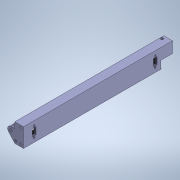
# Autodesk Inventor part: slide rail
Saved by Autodesk Inventor 2020 (Build 240168000, 168)
## iProperties
Created: 2026-07-07
Part Number: slide rail
Material: Steel
Document SubType Name: Modeling
Designer: drago
Density: 7.85 g/cm^3
Appearance: Slate Blue
Author: drago
Autodesk Inventor part; units mm, degrees
ref_plane "YZ Plane" through (0, 0, 0) normal (1, 0, 0) x (0, 1, 0)
ref_plane "XZ Plane" through (0, 0, 0) normal (0, 1, 0) x (-1, 0, 0)
ref_plane "XY Plane" through (0, 0, 0) normal (0, 0, 1) x (1, 0, 0)
sketch "Sketch1" plane through (0, 0, 0) normal (0, 0, 1) x (1, 0, 0)
  line L0 (-0.5, -2.9) -> (6.5, -2.9)
  line L1 (6.5, -2.9) -> (6.5, 12.9)
  line L2 (6.5, 12.9) -> (-0.5, 12.9)
  line L3 (-0.5, 14.9) -> (8.5, 14.9)
  line L4 (8.5, 14.9) -> (8.5, -4.9)
  line L5 (8.5, -4.9) -> (-0.5, -4.9)
  line L6 (-0.5, 12.9) -> (-0.5, 14.9)
  line L7 (-0.5, -4.9) -> (-0.5, -2.9)
  circle A0 centre (-5, 5) radius 1.45
  circle A1 centre (-5, 5) radius 1.45
  circle A2 centre (-5, 5) radius 4
  point P0 (0, 0)
  constraints: 16 end point, 3 centre point, 3 perpendicular, 2 coincident, 2 parallel, 1 horizontal, 2 other
extrude "Extrusion1" add sketch "Sketch1" along normal blind 180
extrude "Extrusion2" cut sketch "Sketch1" along normal blind 160 contours A2
extrude "Extrusion3" add sketch "Sketch1" along normal blind 20 contours A2
sketch "Sketch2" plane through (-0.5, 14.9, 0) normal (0, 1, 0) x (1, 0, 0)
  line L0 (9, 0) -> (0, 0) projected
  line L1 (0, 0) -> (0, -180) projected
  line L2 (9, -180) -> (0, -180) projected
  line L3 (9, 0) -> (9, -180) projected
  point P0 (0.5, 0)
extrude "Extrusion4" add sketch "Sketch2" along normal blind 1
sketch "Sketch3" plane through (-0.5, -4.9, 0) normal (0, -1, 0) x (1, 0, 0)
  line L0 (0, 0) -> (9, 0) projected
  line L1 (9, 0) -> (9, 180) projected
  line L2 (0, 180) -> (9, 180) projected
  line L3 (0, 0) -> (0, 180) projected
  point P0 (0.5, 0)
extrude "Extrusion5" add sketch "Sketch3" along normal blind 1
sketch "Sketch4" plane through (8.5, 15.9, 180) normal (1, 0, 0) x (0, 0, -1)
  line L0 (180, 0) -> (180, -21.8) projected
  line L1 (0, 0) -> (180, 0) projected
  line L2 (0, 0) -> (0, -21.8) projected
  line L3 (180, -21.8) -> (0, -21.8) projected
  point P0 (180, -15.9)
extrude "Extrusion6" add sketch "Sketch4" along normal blind 1
sketch "Sketch5" plane through (-5, 5, 0) normal (0, 0, -1) x (-1, 0, 0)
  circle A0 centre (0, 0) radius 1.45 projected
  point P0 (-5, -5)
extrude "Extrusion7" add sketch "Sketch5" against normal blind 14
sketch "Sketch6" plane through (-5, 5, 180) normal (0, 0, 1) x (1, 0, 0)
  circle A0 centre (0, 0) radius 1.45 projected
  point P0 (5, -5)
extrude "Extrusion8" add sketch "Sketch6" against normal blind 14
sketch "Sketch7" plane through (-5, 5, 0) normal (0, 0, -1) x (-1, 0, 0)
  line L0 (-4.5, 7.9) -> (-4.5, 10.9) projected
  line L1 (-4.5, 10.9) -> (2.9603, 2.69)
  circle A0 centre (0, 0) radius 4 projected
  line L2 (-4.5, -7.9) -> (-4.5, -10.9) projected
  line L3 (-4.5, -10.9) -> (2.9603, -2.69)
  line L4 (-4.5, 7.9) -> (-11.5, 7.9) projected
  line L5 (-4.5, -7.9) -> (-4.5, -10.9) projected
  line L6 (-11.5, -7.9) -> (-4.5, -7.9) projected
  line L7 (-11.5, 7.9) -> (-11.5, -7.9) projected
  line L8 (-4.5, 7.9) -> (-11.5, 7.9) projected
  line L9 (-4.5, 7.9) -> (-4.5, 10.9) projected
  line L10 (-4.5, 10.9) -> (-14.5, 10.9) projected
  line L11 (-14.5, -10.9) -> (-14.5, 10.9) projected
  line L12 (-4.5, -10.9) -> (-14.5, -10.9) projected
  point P0 (-5, -5)
  point P1 (2.9603, -2.69)
  constraints: 4 end point, 4 other
extrude "Extrusion9" add sketch "Sketch7" against normal blind 18 contours L0 L1 A0 L3 L2 L6 L7 L4
sketch "Sketch8" plane through (-0.5, 12.9, 18) normal (-1, 0, 0) x (0, 0, 1)
  line L0 (0, 3) -> (0, 0) projected
  line L1 (0, 3) -> (-5, 3)
  line L2 (-5, 3) -> (-5, -3.9)
  line L3 (-5, -3.9) -> (0, -3.9)
  line L4 (0, -3.9) -> (0, 3)
  point P0 (-18, -12.9)
  dimension "d19" = 5
  constraints: 8 end point, 2 parallel, 1 horizontal, 1 perpendicular
  measures "d19" distance of L3.end L2.end
extrude "Extrusion10" cut sketch "Sketch8" along normal blind 18
sketch "Sketch9" plane through (-5, 5, 180) normal (0, 0, 1) x (1, 0, 0)
  line L0 (4.5, -7.9) -> (4.5, -10.9) projected
  line L1 (4.5, -10.9) -> (-2.9603, -2.69)
  arc A0 (0, 4) -> (-2.9603, 2.69) centre (0, 0) ccw projected
  line L2 (4.5, 10.9) -> (-2.9603, 2.69)
  line L3 (4.5, 7.9) -> (4.5, 4) projected
  line L4 (4.5, 4) -> (0, 4) projected
  arc A1 (-2.9603, -2.69) -> (0, 4) centre (0, 0) ccw projected
  line L5 (-2.9603, -2.69) -> (4.5, -10.9) projected
  line L6 (4.5, -7.9) -> (4.5, -10.9) projected
  line L7 (11.5, -7.9) -> (4.5, -7.9) projected
  line L8 (11.5, 7.9) -> (11.5, -7.9) projected
  line L9 (4.5, 7.9) -> (11.5, 7.9) projected
  line L10 (-1.77, 4) -> (4.5, 10.9) projected
  line L11 (4.5, 7.9) -> (4.5, 10.9) projected
  point P0 (5, -5)
  constraints: 4 end point, 1 tangent
extrude "Extrusion11" add sketch "Sketch9" against normal blind 18
sketch "Sketch10" plane through (-0.5, 9, 13) normal (-1, 0, 0) x (0, 0, 1)
  line L0 (149, 3.9) -> (149, 6.9) projected
  line L1 (149, 6.9) -> (154, 6.9)
  line L2 (154, 6.9) -> (154, 0)
  line L3 (154, 0) -> (149, 0)
  line L4 (149, 0) -> (149, 6.9)
  point P0 (-13, -9)
  dimension "d24" = 5
  constraints: 8 end point, 2 parallel, 1 horizontal, 1 perpendicular
  measures "d24" distance of L2.end L3.end
extrude "Extrusion12" cut sketch "Sketch10" along normal blind 18
sketch "Sketch12" plane through (-0.5, -5.9, 0) normal (0, -1, 0) x (1, 0, 0)
  line L0 (-5.95, 20) -> (-3.05, 20) projected
  circle A0 centre (2, 4) radius 1.4
  circle A1 centre (2, 4) radius 9.5
  point P0 (0.5, 0)
  dimension "d42" = 19
  constraints: 2 centre point, 1 coincident
  measures "d42" diameter of A1
extrude "Extrusion13" cut sketch "Sketch12" against normal blind 9
extrude "Extrusion14" cut sketch "Sketch12" against normal blind 23 contours A0
sketch "Sketch13" plane through (-0.5, 9, 13) normal (-1, 0, 0) x (0, 0, 1)
  line L0 (149, 0) -> (149, 3.9) projected
  line L1 (149, 0) -> (153.7, 0)
  line L2 (149, 3.2) -> (149, 0)
  line L3 (-13, 6.9) -> (167, 6.9) projected
  line L4 (149, 0) -> (159, 0)
  line L5 (159, 0) -> (159, 6.9)
  line L6 (159, 6.9) -> (149, 6.9)
  line L7 (149, 6.9) -> (149, 0)
  line L8 (5, 3.9) -> (5, 0) projected
  line L9 (5, 0) -> (-5, 0)
  line L10 (-5, 0) -> (-5, 6.9)
  line L11 (-5, 6.9) -> (5, 6.9)
  line L12 (5, 6.9) -> (5, 0)
  line L13 (5, 0) -> (0.3, 0)
  line L14 (5, 3.2) -> (5, 0)
  circle A0 centre (2.3, 3.2) radius 0.9
  circle A1 centre (151.7, 3.2) radius 0.9
  point P0 (-13, -9)
  point P1 (153.7, 0)
  dimension "d49" = 10
  dimension "d50" = 10
  constraints: 24 end point, 4 horizontal, 4 parallel, 2 centre point, 2 perpendicular, 2 point on line
  measures "d49" distance of L6.end L5.end
  measures "d50" distance of L10.end L11.end
extrude "Extrusion15" cut sketch "Sketch13" along normal blind 10 contours L0 L7 L3 L5 L4 L1 | L3 L12 L8 L9 L10 | A0 | A1
sketch "Sketch14" plane through (9.5, 15.9, 180) normal (1, 0, 0) x (0, 0, -1)
  line L0 (0, -21.8) -> (170.8765, -21.8) projected
  line L1 (0, 0) -> (8, 0)
  line L2 (8, 0) -> (8, -21.8)
  line L3 (8, -21.8) -> (0, -21.8)
  line L4 (0, -21.8) -> (0, 0)
  point P0 (180, -15.9)
  dimension "d60" = 8
  constraints: 8 end point, 2 parallel, 1 horizontal, 1 perpendicular, 1 point on line
  measures "d60" distance of L2.end L3.end
extrude "Extrusion17" cut sketch "Sketch14" against normal blind 20
sketch "Sketch15" plane through (9.5, -5.9, 172) normal (0, 0, 1) x (1, 0, 0)
  circle A0 centre (-14.5, 10.9) radius 1.45 projected
  circle A1 centre (-14.5, 10.9) radius 1.45
  point P0 (-9.5, 5.9)
  constraints: 1 centre point, 1 coincident
extrude "Extrusion18" cut sketch "Sketch15" against normal blind 20
sketch "Sketch16" plane through (-0.5, 3.1, 0) normal (0, -1, 0) x (1, 0, 0)
  line L0 (-8.5, 0) -> (-8.5, 20) projected
  line L1 (-8.5, 0) -> (-1.5, 0)
  line L2 (-1.5, 0) -> (-1.5, 10)
  line L3 (-1.5, 10) -> (-8.5, 10)
  line L4 (-8.5, 10) -> (-8.5, 0)
  point P0 (0.5, 0)
  dimension "d65" = 7
  dimension "d66" = 10
  constraints: 8 end point, 2 parallel, 1 horizontal, 1 perpendicular, 1 point on line
  measures "d65" distance of L3.end L2.end
  measures "d66" distance of L2.end L1.end
extrude "Extrusion19" cut sketch "Sketch16" along normal mid plane 30
sketch "Sketch17" plane through (-2, 3.1, 10) normal (0, 0, -1) x (-1, 0, 0)
  circle A0 centre (3, 1.9) radius 1.45 projected
  circle A1 centre (3, 1.9) radius 1.45
  point P0 (-2, -3.1)
  constraints: 1 centre point, 1 coincident
extrude "Extrusion20" cut sketch "Sketch17" against normal blind 30
sketch "Sketch18" plane through (-2, 3.1, 10) normal (0, 0, -1) x (-1, 0, 0)
  line L0 (0, 5.9) -> (0, 0) projected
  line L1 (0, 5.9) -> (8.7441, 5.9)
  line L2 (8.7441, 5.9) -> (8.7441, -5.7339)
  line L3 (8.7441, -5.7339) -> (0, -5.7339)
  line L4 (0, -5.7339) -> (0, 5.9)
  point P0 (-2, -3.1)
  constraints: 8 end point, 2 parallel, 1 horizontal, 1 perpendicular
extrude "Extrusion21" cut sketch "Sketch18" against normal blind 2
fillet "Fillet1" radius 2 1 edges at (9.5, -1.4, 9.1235)
sketch "Sketch19" plane through (9.5, -5.9, 172) normal (0, 0, 1) x (1, 0, 0)
  circle A0 centre (-14.5, 10.9) radius 1.45 projected
  circle A1 centre (-14.5, 10.9) radius 4
  line L0 (-10, 14.9) -> (-16.27, 14.9) projected
  line L1 (-16.27, 14.9) -> (-17.4603, 13.59)
  line L2 (-17.4603, 13.59) -> (-16.27, 14.9) projected
  point P0 (-9.5, 5.9)
  point P1 (-14.5, 14.9)
  constraints: 2 end point, 1 coincident, 1 collinear, 1 horizontal, 1 point on line, 3 other
extrude "Extrusion22" cut sketch "Sketch19" against normal blind 300 contours L1 L0 A1
sketch "Sketch21" plane through (9.5, -5.9, 172) normal (0, 0, 1) x (1, 0, 0)
  circle A0 centre (-3, 3) radius 0.9
  circle A1 centre (-9, 3) radius 0.9
  point P0 (0, 0)
  constraints: 2 centre point, 1 coincident
extrude "Extrusion23" cut sketch "Sketch21" against normal blind 8
sketch "Sketch22" plane through (9.5, -5.9, 172) normal (0, 0, 1) x (1, 0, 0)
  circle A0 centre (-3, 19) radius 0.9
  point P0 (-9.5, 5.9)
  constraints: 1 centre point
extrude "Extrusion24" cut sketch "Sketch22" against normal blind 8
chamfer "Chamfer2" distance 0.5 angle 45 3 edges at (-0.4, -2.9, 172) (5.6, -2.9, 172) (5.6, 13.1, 172)
chamfer "Chamfer3" distance 0.75 angle 45 3 edges at (-3.55, 5, 20) (-6.45, 5, 160) (-3.55, 5, 12)
sketch "Sketch23" plane through (6.5, -2.9, 18) normal (-1, 0, 0) x (0, 0, 1)
  line L0 (0, 3.9) -> (2, 3.9) projected
  line L1 (0, 3.9) -> (4, 3.9)
  line L2 (4, 3.9) -> (4, 11.9)
  line L3 (4, 11.9) -> (0, 11.9)
  line L4 (0, 11.9) -> (0, 3.9)
  line L5 (142, 3.9) -> (144, 3.9) projected
  line L6 (144, 3.9) -> (140, 3.9)
  line L7 (140, 3.9) -> (140, 11.9)
  line L8 (140, 11.9) -> (144, 11.9)
  line L9 (144, 11.9) -> (144, 3.9)
  point P0 (-18, 2.9)
  dimension "d93" = 4
  dimension "d94" = 4
  constraints: 16 end point, 4 parallel, 2 horizontal, 2 perpendicular, 2 point on line
  measures "d93" distance of L3.end L2.end
  measures "d94" distance of L7.end L8.end
extrude "Extrusion25" cut sketch "Sketch23" against normal blind 8
sketch "Sketch24" plane through (6.5, -2.9, 18) normal (-1, 0, 0) x (0, 0, 1)
  line L0 (0, 0) -> (144, 0) projected
  line L1 (0, 5.21) -> (0, -3) projected
  circle A0 centre (2, 2) radius 1
  line L2 (2, 5.7) -> (2, 10.1) projected
  circle A1 centre (2, 13.8) radius 1
  line L3 (0, 0) -> (144, 0) projected
  circle A2 centre (142, 2) radius 1
  circle A3 centre (142, 13.8) radius 1
  point P0 (-18, 2.9)
  dimension "d98" = 2
  constraints: 4 centre point
  measures "d98" diameter of A0
extrude "Extrusion26" cut sketch "Sketch24" against normal blind 10
sketch "Sketch25" plane through (-0.5, 9, 18) normal (-1, 0, 0) x (0, 0, 1)
  line L0 (0, 3.9) -> (144, 3.9) projected
  line L1 (0, 3.9) -> (144, 3.9)
  line L2 (144, 3.9) -> (144, 4.05)
  line L3 (144, 4.05) -> (0, 4.05)
  line L4 (0, 4.05) -> (0, 3.9)
  line L5 (0, -11.9) -> (144, -11.9) projected
  line L6 (144, -14.9) -> (144, -11.9) projected
  line L7 (0, -11.9) -> (144, -11.9)
  line L8 (144, -11.9) -> (144, -12.05)
  line L9 (144, -12.05) -> (0, -12.05)
  line L10 (0, -12.05) -> (0, -11.9)
  point P0 (-18, -9)
  dimension "d102" = 0.15
  constraints: 16 end point, 4 parallel, 2 horizontal, 2 perpendicular, 1 point on line
  measures "d102" distance of L7.end L8.end
extrude "Extrusion27" cut sketch "Sketch25" against normal up to surface (7 mm away)
sketch "Sketch26" plane through (6.5, 1, 22) normal (-1, 0, 0) x (0, 0, 1)
  circle A0 centre (-2, -1.9) radius 1 projected
  circle A1 centre (138, 9.9) radius 1 projected
  circle A2 centre (-2, 9.9) radius 1 projected
  circle A3 centre (138, -1.9) radius 1 projected
  line L0 (-4, 8) -> (0, 8) projected
  line L1 (0, 8) -> (0, 0) projected
  line L2 (0, 0) -> (-4, 0) projected
  line L3 (-4, -4.05) -> (-4, 0) projected
  line L4 (140, -4.05) -> (-4, -4.05) projected
  line L5 (140, -4.05) -> (140, 0) projected
  line L6 (140, 0) -> (136, 0) projected
  line L7 (136, 0) -> (136, 8) projected
  line L8 (136, 8) -> (140, 8) projected
  line L9 (140, 8) -> (140, 12.05) projected
  line L10 (-4, 12.05) -> (140, 12.05) projected
  line L11 (-4, 12.05) -> (-4, 8) projected
  point P0 (-22, -1)
extrude "Extrusion28" cut sketch "Sketch26" against normal blind 0.75
sketch "Sketch27" plane through (-0.5, 13.05, 18) normal (0, -1, 0) x (1, 0, 0)
  line L0 (0, 144) -> (7.75, 144) projected
  line L1 (0, 0) -> (0, 144) projected
  line L2 (0, 0) -> (7.75, 0) projected
  line L3 (7.75, 0) -> (7.75, 144) projected
  point P0 (0.5, -18)
extrude "Extrusion29" add sketch "Sketch27" along normal blind 0.09
sketch "Sketch28" plane through (-0.5, -3.05, 162) normal (0, 1, 0) x (1, 0, 0)
  line L0 (0, 144) -> (7.75, 144) projected
  line L1 (0, 0) -> (0, 144) projected
  line L2 (0, 0) -> (7.75, 0) projected
  line L3 (7.75, 0) -> (7.75, 144) projected
  point P0 (0.5, 162)
extrude "Extrusion30" add sketch "Sketch28" along normal blind 0.09
extrude "Extrusion31" cut sketch "Sketch13" against normal blind 6 contours A0 | A1
chamfer "Chamfer4" distance 0.5 angle 45 2 edges at (-0.5, 12.2, 14.4) (-0.5, 12.2, 163.8)
body "Solid1"
